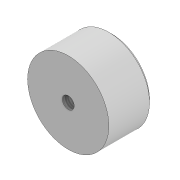
# Autodesk Inventor part: Gummistopl klein
Saved by Autodesk Inventor 2020 (Build 240168000, 168)
## iProperties
Created: 2021-06-23
Part Number: Gummistopl klein
Material: Generisch
Document SubType Name: Modeling
Designer: mike8
Density: 1 g/cm^3
Appearance: Vorgabe
Author: mike8
Autodesk Inventor part; units mm, degrees
ref_plane "YZ Plane" through (0, 0, 0) normal (1, 0, 0) x (0, 1, 0)
ref_plane "XZ Plane" through (0, 0, 0) normal (0, 1, 0) x (-1, 0, 0)
ref_plane "XY Plane" through (0, 0, 0) normal (0, 0, 1) x (1, 0, 0)
sketch "Skizze1" plane through (0, 0, 0) normal (0, 0, 1) x (1, 0, 0)
  line L0 (-19.6, 0) -> (19.6, 0) projected
  line L1 (0, -19.6) -> (0, 19.6) projected
  circle A0 centre (0, 0) radius 14
  dimension "d0" = 28
  constraints: 1 centre point, 1 coincident
  measures "d0" diameter of A0
extrude "Extrusion1" add sketch "Skizze1" along normal blind 15
chamfer "Fase1" distance 1 angle 45 1 edges at (-14, 0, 0)
sketch "Skizze2" plane through (0, 0, 15) normal (0, 0, 1) x (1, 0, 0)
  point P0 (0, 0)
  point P1 (0, 0)
  constraints: 1 coincident
hole "Bohrung1" at (0, 0, 15) direction (0, 0, -1) diameter 4.134 depth 11 tip angle 118 thread size "M5x0.8" class "6H" standard "ISO Metric profile"
